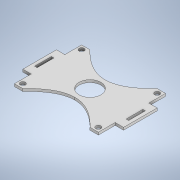
# Autodesk Inventor part: bottomBearingHolder
Saved by Autodesk Inventor 2020 (Build 240168000, 168)
## iProperties
Created: 2019-06-18
Part Number: bottomBearingHolder
Material: Generic
Document SubType Name: Modeling
Designer: Vivek Muskan
Density: 1 g/cm^3
Appearance: Default
Author: Vivek Muskan
Autodesk Inventor part; units mm, degrees
ref_plane "YZ Plane" through (0, 0, 0) normal (1, 0, 0) x (0, 1, 0)
sketch "Sketch1" plane through (0, 0, 0) normal (0, 1, 0) x (-1, 0, 0)
  circle A0 centre (0, 0) radius 6.5
  line L0 (25, 20) -> (-25, 20)
  line L1 (-25, 20) -> (-25, -20)
  line L2 (-25, -20) -> (25, -20)
  line L3 (25, -20) -> (25, 20)
  line L4 (25, 20) -> (-25, -20) construction
  line L5 (-25, 20) -> (25, -20) construction
  line L6 (-25, 0) -> (-30, 0)
  line L7 (-30, 0) -> (-30, -10)
  line L8 (-30, -10) -> (-25, -10)
  line L9 (-25, -10) -> (-25, 0)
  line L10 (-30, 0) -> (-25, 0)
  line L11 (-25, 0) -> (-25, 10)
  line L12 (-25, 10) -> (-30, 10)
  line L13 (-30, 10) -> (-30, 0)
  line L14 (-25, 10) -> (-25, 5)
  line L15 (-25, 5) -> (-26.5, 5)
  line L16 (-26.5, 5) -> (-28, 5)
  line L17 (-28, 5) -> (-28, -5)
  line L18 (-28, -5) -> (-26.5, -5)
  line L19 (-26.5, -5) -> (-26.5, 5)
  line L20 (0, 0) -> (0, -20)
  line L21 (30, 0) -> (30, -10)
  line L22 (30, -10) -> (25, -10)
  line L23 (26.5, -5) -> (26.5, 5)
  line L24 (28, 5) -> (28, -5)
  line L25 (28, -5) -> (26.5, -5)
  line L26 (26.5, 5) -> (28, 5)
  line L27 (25, 10) -> (30, 10)
  line L28 (30, 10) -> (30, 0)
  dimension "d0" = 13
  dimension "d1" = 50
  dimension "d2" = 40
  dimension "d3" = 5
  dimension "d4" = 10
  dimension "d5" = 5
  dimension "d6" = 10
  dimension "d7" = 5
  dimension "d8" = 1.5
  dimension "d9" = 1.5
  dimension "d10" = 10
  constraints: 58 end point, 9 symmetric about line, 8 parallel, 5 perpendicular, 4 horizontal, 4 midpoint, 1 centre point, 1 coincident
  measures "d0" diameter of A0
  measures "d1" distance of L2.end L1.end
  measures "d2" distance of L1.end L0.end
  measures "d3" distance of L8.end L7.end
  measures "d4" distance of L7.end L6.end
  measures "d5" distance of L12.end L11.end
  measures "d6" distance of L12.end L6.end
  measures "d7" distance of L11.end L15.start
  measures "d8" distance of L15.start L15.end
  measures "d9" distance of L19.start L17.end
  measures "d10" distance of L17.end L17.start
extrude "Extrusion1" add sketch "Sketch1" along normal blind 1.5 contours L2 L1 L0 L3 | L8 L7 L6 L17 L18 L19 L1 | L3 L27 L28 L21 L22 | L6 L19 L15 L1 | L15 L16 L17 L6 L13 L12 L1
sketch "Sketch2" plane through (0, 1.5, 0) normal (0, 1, 0) x (1, 0, 0)
  line L0 (0, 0) -> (22.5, 0)
  line L1 (22.5, 0) -> (22.5, 17.5)
  line L2 (25, 20) -> (-25, 20) projected
  circle A0 centre (22.5, 17.5) radius 1.5
  dimension "d13" = 22.5
  dimension "d14" = 17.5
  dimension "d15" = 3
  constraints: 4 end point, 1 centre point, 1 coincident, 1 horizontal, 1 perpendicular
  measures "d13" distance of L0.start L0.end
  measures "d14" distance of L0.end L1.end
  measures "d15" diameter of A0
extrude "Extrusion2" cut sketch "Sketch2" against normal blind 1.5
ref_plane "Work Plane1" through (0, 0, 20) normal (1, 0, 0) x (0, 0, -1)
ref_plane "Work Plane2" through (-25, 0, 0) normal (0, 0, 1) x (1, 0, 0)
mirror "Mirror1" about plane through (0, 0, 20) normal (1, 0, 0) of "Extrusion2"
mirror "Mirror2" about plane through (-25, 0, 0) normal (0, 0, 1) of "Extrusion2", "Mirror1"
sketch "Sketch3" plane through (0, 1.5, 0) normal (0, 1, 0) x (1, 0, 0)
  line L0 (25, 10) -> (25, 20) projected
  line L1 (25, 20) -> (20, 20)
  line L2 (25, 20) -> (-25, 20) projected
  line L3 (0, 0) -> (0, 9)
  line L4 (20, 20) -> (9.6256, 9) construction
  line L5 (9.6256, 9) -> (0, 9) construction
  spline S0 degree 2 poles (20, 20) (9.6256, 9) (0, 9) knots 1 1 1 2 2 2
  line L6 (0, 0) -> (9.6256, 0)
  line L7 (-20, 20) -> (-9.6256, 9) construction
  line L8 (-9.6256, 9) -> (0, 9) construction
  spline S1 degree 2 poles (-20, 20) (-9.6256, 9) (0, 9) knots 1 1 1 2 2 2
  line L9 (20, -20) -> (9.6256, -9) construction
  line L10 (9.6256, -9) -> (0, -9) construction
  spline S2 degree 2 poles (20, -20) (9.6256, -9) (0, -9) knots 1 1 1 2 2 2
  line L11 (-20, -20) -> (-9.6256, -9) construction
  spline S3 degree 2 poles (-20, -20) (-9.6256, -9) (0, -9) knots 1 1 1 2 2 2
  line L12 (-9.6256, -9) -> (0, -9) construction
  line L13 (20, 20) -> (-20, 20)
  line L14 (20, -20) -> (-20, -20)
  line L15 (-25, -20) -> (25, -20) projected
  dimension "d18" = 5
  dimension "d19" = 9
  constraints: 10 end point, 7 symmetric about line, 2 collinear, 1 horizontal, 1 parallel, 1 point on line, 1 vertical, 12 other
  measures "d18" distance of L0.end L1.end
  measures "d19" distance of L3.start L3.end
extrude "Extrusion3" cut sketch "Sketch3" against normal blind 1.5
body "Solid1"
